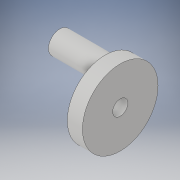
# Autodesk Inventor part: SpoolWinderHandle
Saved by Autodesk Inventor 2019 (Build 230136000, 136)
## iProperties
Created: 2019-01-14
Part Number: SpoolWinderHandle
Material: Generic
Document SubType Name: Modeling
Designer: Kepler
Density: 1 g/cm^3
Appearance: Default
Author: Kepler
Autodesk Inventor part; units mm, degrees
ref_plane "YZ Plane" through (0, 0, 0) normal (1, 0, 0) x (0, 1, 0)
ref_plane "XZ Plane" through (0, 0, 0) normal (0, 1, 0) x (-1, 0, 0)
ref_plane "XY Plane" through (0, 0, 0) normal (0, 0, 1) x (1, 0, 0)
sketch "Sketch1" plane through (0, 0, 0) normal (0, 0, 1) x (1, 0, 0)
  line L0 (0, 0) -> (0, 20)
  line L1 (0, 20) -> (10, 20)
  line L2 (10, 20) -> (10, 0)
  line L3 (10, 0) -> (0, 0)
  line L4 (0, 25) -> (10, 25)
  dimension "d1" = 20
  dimension "d2" = 10
  dimension "d3" = 5
  dimension "d4" = 10
  dimension "d5" = 10
  constraints: 10 end point, 3 perpendicular, 1 parallel, 1 vertical
  measures "d1" distance of L0.start L0.end
  measures "d2" distance of L0.end L1.end
  measures "d3" distance of L0.end L4.start
  measures "d4" distance of L4.start L4.end
  measures "d5" diameter of L1 L4
revolve "Revolution1" add sketch "Sketch1" angle 360 about axis through (0, 25, 0) along (1, 0, 0)
sketch "Sketch2" plane through (0, 25, 0) normal (-1, 0, 0) x (0, 0, 1)
  circle A0 centre (0, 17.5) radius 7.5
  circle A1 centre (0, 0) radius 25 projected
  point P0 (0, -25)
  dimension "d7" = 15
  constraints: 1 centre point, 1 vertical alignment, 1 other
  measures "d7" diameter of A0
extrude "Extrusion1" add sketch "Sketch2" along normal blind 30 contours A0
body "Solid1"
